Autodesk Inventor part; units mm, degrees
(part 2 of 2)
sketch "Sketch18" plane through (0, 0, -0.2) normal (0, 0, -1) x (-1, 0, 0)
  line L0 (-13.9597, 17.5749) -> (-9.7521, 15.1456) projected
  line L1 (-9.7521, 15.1456) -> (-5.5444, 17.5749) projected
  line L2 (-5.5444, 17.5749) -> (-5.5444, 22.4335) projected
  line L3 (-5.5444, 22.4335) -> (-9.7521, 24.8628) projected
  line L4 (-9.7521, 24.8628) -> (-13.9597, 22.4335) projected
  line L5 (-13.9597, 22.4335) -> (-13.9597, 17.5749) projected
  line L6 (-34.8886, 65.4022) -> (-34.8886, 72.3894) projected
  line L7 (-34.8886, 72.3894) -> (-40.9397, 75.883) projected
  line L8 (-40.9397, 75.883) -> (-46.9908, 72.3894) projected
  line L9 (-46.9908, 72.3894) -> (-46.9908, 65.4022) projected
  line L10 (-46.9908, 65.4022) -> (-40.9397, 61.9086) projected
  line L11 (-40.9397, 61.9086) -> (-34.8886, 65.4022) projected
  line L12 (-49.5403, 66.4665) -> (-49.5403, 71.3251) projected
  line L13 (-49.5403, 71.3251) -> (-53.7479, 73.7544) projected
  line L14 (-53.7479, 73.7544) -> (-57.9556, 71.3251) projected
  line L15 (-57.9556, 71.3251) -> (-57.9556, 66.4665) projected
  line L16 (-57.9556, 66.4665) -> (-53.7479, 64.0372) projected
  line L17 (-53.7479, 64.0372) -> (-49.5403, 66.4665) projected
  line L18 (0, 0) -> (-63.5, 0)
  line L19 (-63.5, 0) -> (-63.5, 88.9)
  line L20 (-63.5, 88.9) -> (0, 88.9)
  line L21 (0, 88.9) -> (0, 0)
  line L22 (-40.9397, 26.9914) -> (-46.9908, 23.4978) projected
  line L23 (-46.9908, 23.4978) -> (-46.9908, 16.5106) projected
  line L24 (-46.9908, 16.5106) -> (-40.9397, 13.017) projected
  line L25 (-40.9397, 13.017) -> (-34.8886, 16.5106) projected
  line L26 (-34.8886, 16.5106) -> (-34.8886, 23.4978) projected
  line L27 (-34.8886, 23.4978) -> (-40.9397, 26.9914) projected
  line L28 (-22.5603, 13.017) -> (-16.5092, 16.5106) projected
  line L29 (-16.5092, 16.5106) -> (-16.5092, 23.4978) projected
  line L30 (-16.5092, 23.4978) -> (-22.5603, 26.9914) projected
  line L31 (-22.5603, 26.9914) -> (-28.6114, 23.4978) projected
  line L32 (-28.6114, 23.4978) -> (-28.6114, 16.5106) projected
  line L33 (-28.6114, 16.5106) -> (-22.5603, 13.017) projected
  line L34 (-24.4329, 66.1976) -> (-24.4329, 72.4542) projected
  line L35 (-22.5603, 61.9086) -> (-16.5092, 65.4022) projected
  line L36 (-16.5092, 65.4022) -> (-16.5092, 72.3894) projected
  line L37 (-16.5092, 72.3894) -> (-22.5603, 75.883) projected
  line L38 (-22.5603, 75.883) -> (-28.6114, 72.3894) projected
  line L39 (-28.6114, 72.3894) -> (-28.6114, 65.4022) projected
  line L40 (-28.6114, 65.4022) -> (-22.5603, 61.9086) projected
  line L41 (-34.8886, 40.9564) -> (-34.8886, 47.9436) projected
  line L42 (-34.8886, 47.9436) -> (-40.9397, 51.4372) projected
  line L43 (-40.9397, 51.4372) -> (-46.9908, 47.9436) projected
  line L44 (-46.9908, 47.9436) -> (-46.9908, 40.9564) projected
  line L45 (-46.9908, 40.9564) -> (-40.9397, 37.4628) projected
  line L46 (-40.9397, 37.4628) -> (-34.8886, 40.9564) projected
  line L47 (-28.6114, 47.9436) -> (-28.6114, 40.9564) projected
  line L48 (-22.5603, 37.4628) -> (-16.5092, 40.9564) projected
  line L49 (-16.5092, 40.9564) -> (-16.5092, 47.9436) projected
  line L50 (-16.5092, 47.9436) -> (-22.5603, 51.4372) projected
  line L51 (-22.5603, 51.4372) -> (-28.6114, 47.9436) projected
  line L52 (-28.6114, 40.9564) -> (-22.5603, 37.4628) projected
  line L53 (-31.75, 49.6857) -> (-25.6989, 53.1793) projected
  line L54 (-25.6989, 53.1793) -> (-25.6989, 60.1665) projected
  line L55 (-25.6989, 60.1665) -> (-31.75, 63.6601) projected
  line L56 (-31.75, 63.6601) -> (-37.8011, 60.1665) projected
  line L57 (-37.8011, 60.1665) -> (-37.8011, 53.1793) projected
  line L58 (-37.8011, 53.1793) -> (-31.75, 49.6857) projected
  line L59 (-31.75, 25.2399) -> (-25.6989, 28.7335) projected
  line L60 (-25.6989, 28.7335) -> (-25.6989, 35.7207) projected
  line L61 (-25.6989, 35.7207) -> (-31.75, 39.2143) projected
  line L62 (-31.75, 39.2143) -> (-37.8011, 35.7207) projected
  line L63 (-37.8011, 35.7207) -> (-37.8011, 28.7335) projected
  line L64 (-37.8011, 28.7335) -> (-31.75, 25.2399) projected
  spline S0 degree 2 poles (-52.0272, 83.2599) (-52.0272, 82.6424) (-52.4471, 81.6791) (-53.0399, 81.2262) knots 0 0 0 0.5 1 1 1 projected
  spline S1 degree 2 poles (-53.0399, 81.2262) (-53.3939, 81.3415) (-54.2666, 81.745) (-54.4725, 81.8602) knots 0 0 0 0.5 1 1 1 projected
  spline S2 degree 2 poles (-54.4725, 81.8602) (-54.9582, 82.1402) (-55.444, 82.84) (-55.444, 83.3422) knots 0 0 0 0.5 1 1 1 projected
  spline S3 degree 2 poles (-55.444, 83.3422) (-55.444, 84.0421) (-54.4972, 84.8572) (-53.7562, 84.8572) knots 0 0 0 0.5 1 1 1 projected
  spline S4 degree 2 poles (-53.7562, 84.8572) (-52.9411, 84.8572) (-52.0272, 83.9433) (-52.0272, 83.2599) knots 0 0 0 0.5 1 1 1 projected
  spline S5 degree 2 poles (-51.8378, 78.1717) (-51.8378, 77.2825) (-52.8752, 76.2533) (-53.7315, 76.2533) knots 0 0 0 0.5 1 1 1 projected
  spline S6 degree 2 poles (-53.7315, 76.2533) (-54.5713, 76.2533) (-55.6828, 77.4554) (-55.6828, 78.3775) knots 0 0 0 0.5 1 1 1 projected
  spline S7 degree 2 poles (-55.6828, 78.3775) (-55.6828, 79.0773) (-55.0817, 80.1806) (-54.5219, 80.5511) knots 0 0 0 0.5 1 1 1 projected
  spline S8 degree 2 poles (-54.5219, 80.5511) (-54.0361, 80.3535) (-53.2622, 80.0489) (-53.0316, 79.9171) knots 0 0 0 0.5 1 1 1 projected
  spline S9 degree 2 poles (-53.0316, 79.9171) (-52.3318, 79.5384) (-51.8378, 78.7974) (-51.8378, 78.1717) knots 0 0 0 0.5 1 1 1 projected
  spline S10 degree 2 poles (-56.185, 76.1133) (-55.7487, 75.6934) (-54.5054, 75.2406) (-53.7479, 75.2406) knots 0 0 0 0.5 1 1 1 projected
  spline S11 degree 2 poles (-53.7479, 75.2406) (-52.3318, 75.2406) (-50.4381, 77.0025) (-50.4381, 78.3034) knots 0 0 0 0.5 1 1 1 projected
  spline S12 degree 2 poles (-50.4381, 78.3034) (-50.4381, 79.242) (-51.352, 80.4276) (-52.2412, 80.8393) knots 0 0 0 0.5 1 1 1 projected
  line L65 (-52.2412, 80.8393) -> (-52.2412, 80.8804) projected
  spline S13 degree 2 poles (-52.2412, 80.8804) (-51.492, 81.2592) (-50.6934, 82.593) (-50.6934, 83.2764) knots 0 0 0 0.5 1 1 1 projected
  spline S14 degree 2 poles (-50.6934, 83.2764) (-50.6934, 84.4126) (-52.3647, 85.8616) (-53.7479, 85.8616) knots 0 0 0 0.5 1 1 1 projected
  spline S15 degree 2 poles (-53.7479, 85.8616) (-55.0817, 85.8616) (-56.8108, 84.3302) (-56.8108, 83.1858) knots 0 0 0 0.5 1 1 1 projected
  spline S16 degree 2 poles (-56.8108, 83.1858) (-56.8108, 82.4119) (-56.0862, 81.3744) (-55.337, 80.9381) knots 0 0 0 0.5 1 1 1 projected
  line L66 (-55.337, 80.9381) -> (-55.337, 80.8969) projected
  spline S17 degree 2 poles (-55.337, 80.8969) (-56.1768, 80.4852) (-57.0578, 79.102) (-57.0578, 78.2787) knots 0 0 0 0.5 1 1 1 projected
  spline S18 degree 2 poles (-57.0578, 78.2787) (-57.0578, 77.6447) (-56.6132, 76.525) (-56.185, 76.1133) knots 0 0 0 0.5 1 1 1 projected
  spline S19 degree 2 poles (-11.4728, 5.9847) (-11.4728, 6.6022) (-11.0529, 7.5655) (-10.4601, 8.0183) knots 0 0 0 0.5 1 1 1 projected
  spline S20 degree 2 poles (-10.4601, 8.0183) (-10.1061, 7.9031) (-9.2334, 7.4996) (-9.0275, 7.3844) knots 0 0 0 0.5 1 1 1 projected
  spline S21 degree 2 poles (-9.0275, 7.3844) (-8.5418, 7.1044) (-8.056, 6.4046) (-8.056, 5.9023) knots 0 0 0 0.5 1 1 1 projected
  spline S22 degree 2 poles (-8.056, 5.9023) (-8.056, 5.2025) (-9.0028, 4.3874) (-9.7438, 4.3874) knots 0 0 0 0.5 1 1 1 projected
  spline S23 degree 2 poles (-9.7438, 4.3874) (-10.5589, 4.3874) (-11.4728, 5.3013) (-11.4728, 5.9847) knots 0 0 0 0.5 1 1 1 projected
  spline S24 degree 2 poles (-11.6622, 11.0729) (-11.6622, 11.9621) (-10.6248, 12.9913) (-9.7685, 12.9913) knots 0 0 0 0.5 1 1 1 projected
  spline S25 degree 2 poles (-9.7685, 12.9913) (-8.9287, 12.9913) (-7.8172, 11.7892) (-7.8172, 10.8671) knots 0 0 0 0.5 1 1 1 projected
  spline S26 degree 2 poles (-7.8172, 10.8671) (-7.8172, 10.1672) (-8.4183, 9.064) (-8.9781, 8.6935) knots 0 0 0 0.5 1 1 1 projected
  spline S27 degree 2 poles (-8.9781, 8.6935) (-9.4639, 8.8911) (-10.2378, 9.1957) (-10.4684, 9.3274) knots 0 0 0 0.5 1 1 1 projected
  spline S28 degree 2 poles (-10.4684, 9.3274) (-11.1682, 9.7062) (-11.6622, 10.4472) (-11.6622, 11.0729) knots 0 0 0 0.5 1 1 1 projected
  spline S29 degree 2 poles (-7.315, 13.1313) (-7.7513, 13.5512) (-8.9946, 14.004) (-9.7521, 14.004) knots 0 0 0 0.5 1 1 1 projected
  spline S30 degree 2 poles (-9.7521, 14.004) (-11.1682, 14.004) (-13.0619, 12.2421) (-13.0619, 10.9412) knots 0 0 0 0.5 1 1 1 projected
  spline S31 degree 2 poles (-13.0619, 10.9412) (-13.0619, 10.0026) (-12.148, 8.817) (-11.2588, 8.4053) knots 0 0 0 0.5 1 1 1 projected
  line L67 (-11.2588, 8.4053) -> (-11.2588, 8.3641) projected
  spline S32 degree 2 poles (-11.2588, 8.3641) (-12.008, 7.9854) (-12.8066, 6.6516) (-12.8066, 5.9682) knots 0 0 0 0.5 1 1 1 projected
  spline S33 degree 2 poles (-12.8066, 5.9682) (-12.8066, 4.832) (-11.1353, 3.3829) (-9.7521, 3.3829) knots 0 0 0 0.5 1 1 1 projected
  spline S34 degree 2 poles (-9.7521, 3.3829) (-8.4183, 3.3829) (-6.6892, 4.9143) (-6.6892, 6.0588) knots 0 0 0 0.5 1 1 1 projected
  spline S35 degree 2 poles (-6.6892, 6.0588) (-6.6892, 6.8327) (-7.4138, 7.8701) (-8.163, 8.3065) knots 0 0 0 0.5 1 1 1 projected
  line L68 (-8.163, 8.3065) -> (-8.163, 8.3477) projected
  spline S36 degree 2 poles (-8.163, 8.3477) (-7.3232, 8.7593) (-6.4422, 10.1425) (-6.4422, 10.9659) knots 0 0 0 0.5 1 1 1 projected
  spline S37 degree 2 poles (-6.4422, 10.9659) (-6.4422, 11.5998) (-6.8868, 12.7196) (-7.315, 13.1313) knots 0 0 0 0.5 1 1 1 projected
  constraints: 8 end point, 2 parallel, 1 horizontal, 1 perpendicular, 38 other
extrude "Extrusion21" add sketch "Sketch18" along normal blind 0.4 bodies 3
fillet "Fillet2" radius 3.175 8 edges at (63.5, 0, 0.2) (63.5, 88.9, 0.2) (0, 0, 0.2) (0, 88.9, 0.2) (63.5, 0, -0.3) (63.5, 88.9, -0.3) (0, 0, -0.3) (0, 88.9, -0.3)
